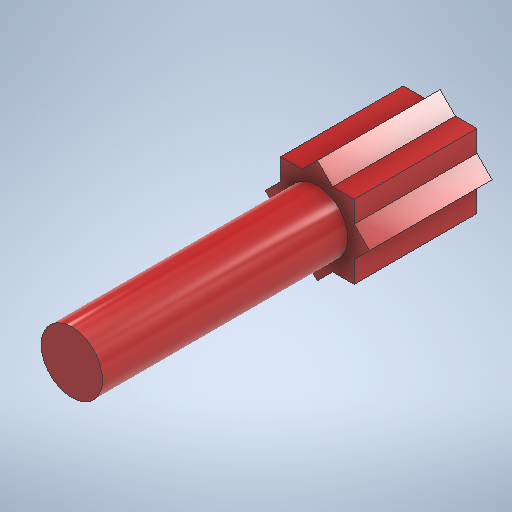
# Autodesk Inventor part: screwhead
Saved by Autodesk Inventor 2025 (Build 290162000, 162)
## iProperties
Created: 2025-05-09
Part Number: screwhead
Material: Generic
Document SubType Name: Modeling
Designer: thesn
Density: 1 g/cm^3
Appearance: Default
Author: thesn
Autodesk Inventor part; units mm, degrees
ref_plane "YZ Plane" through (0, 0, 0) normal (1, 0, 0) x (0, 1, 0)
ref_plane "XZ Plane" through (0, 0, 0) normal (0, 1, 0) x (-1, 0, 0)
ref_plane "XY Plane" through (0, 0, 0) normal (0, 0, 1) x (1, 0, 0)
sketch "Sketch1" plane through (0, 0, 0) normal (0, 0, 1) x (1, 0, 0)
  circle A0 centre (0, 0) radius 0.762
  line L0 (-1.0776, 0) -> (0, 1.0776)
  line L1 (0, 1.0776) -> (1.0776, 0)
  line L2 (1.0776, 0) -> (0, -1.0776)
  line L3 (0, -1.0776) -> (-1.0776, 0)
  line L4 (-0.762, 0.762) -> (0.762, 0.762)
  line L5 (0.762, 0.762) -> (0.762, -0.762)
  line L6 (0.762, -0.762) -> (-0.762, -0.762)
  line L7 (-0.762, -0.762) -> (-0.762, 0.762)
  point P0 (0, 3.175)
  point P1 (-3.175, 0)
  point P2 (-0.898, 0.898)
  point P3 (-0.6286, -0.0898)
  point P4 (-0.5388, -0.5388)
  point P5 (0.5388, -0.5388)
  point P6 (0.3287, 1.2267)
  point P7 (3.7343, 0.7559)
  point P8 (0.5388, 0.5388)
  point P9 (-0.5388, 0.5388)
  point P10 (0, 0.762)
  point P11 (-0.762, 0)
  point P12 (0.3156, 0.762)
  point P13 (-0.3156, 0.762)
  point P14 (-0.762, 0.3156)
  point P15 (-0.762, -0.3156)
  point P16 (-0.3156, -0.762)
  point P17 (0.3156, -0.762)
  point P18 (0.762, -0.3156)
  point P19 (0.762, 0.3156)
  dimension "d0" = 1.524
  dimension "d1" = 1.524
  dimension "d2" = 1.524
  dimension "d3" = 0
  dimension "d12" = 0
  dimension "d13" = 0
  dimension "d16" = 1.524
  dimension "d17" = 1.524
  dimension "d18" = 0
  dimension "d19" = 0
  constraints: 16 end point, 4 parallel, 2 midpoint, 2 perpendicular, 1 centre point, 1 coincident, 1 horizontal
  measures "d0" diameter of A0
  measures "d1" distance of L1.end L2.end
  measures "d2" distance between parallel lines of L2 L0
  measures "d3" horizontal distance of point (0, 0) point (0, 3.175)
  measures "d12" horizontal distance of point (0, 0) L0.end
  measures "d13" vertical distance of point (0, 0) L1.end
  measures "d16" distance of L5.end L6.end
  measures "d17" distance of L4.end L5.end
  measures "d18" horizontal distance of point (0, 0) point (0, 0.762)
  measures "d19" vertical distance of point (0, 0) point (-0.762, 0)
extrude "Extrusion3" add sketch "Sketch1" against normal blind 7.62
sketch "Sketch6" plane through (0, 0, 0) normal (0, 0, 1) x (1, 0, 0)
  line L0 (-0.762, 0.3156) -> (-0.762, 0.762) projected
  circle A0 centre (0, 0) radius 1.0776
  line L1 (-0.762, 0.762) -> (-0.3156, 0.762) projected
  circle A1 centre (0, 0) radius 0.635
  dimension "d33" = 1.27
  constraints: 2 coincident, 1 centre point, 3 other
  measures "d33" diameter of A1
extrude "Extrusion6" cut sketch "Sketch6" against normal blind 5.08
sketch "Sketch7" plane through (0, 0, -7.62) normal (0, 0, -1) x (-1, 0, 0)
  line L0 (-1.6188, 0.635) -> (1.6188, 0.635) construction
  line L1 (1.6188, 0.635) -> (1.6188, -0.635) construction
  line L2 (1.6188, -0.635) -> (-1.6188, -0.635) construction
  line L3 (-1.6188, -0.635) -> (-1.6188, 0.635) construction
  line L4 (-0.1528, -0.1398) -> (-0.1528, -0.2286)
  line L5 (-0.1528, -0.2286) -> (0.0123, -0.2286)
  line L6 (0.0123, -0.2286) -> (0.0123, 0.2282)
  line L7 (0.0123, 0.2282) -> (-0.1657, 0.2282)
  spline S0 degree 2 poles (-0.1657, 0.2282) (-0.2188, 0.2282) (-0.291, 0.1916) (-0.3147, 0.1563) knots 0 0 0 1 2 2 2
  line L8 (-0.3147, 0.1563) -> (-0.5796, -0.2286)
  line L9 (-0.5796, -0.2286) -> (-0.3825, -0.2286)
  line L10 (-0.3825, -0.2286) -> (-0.3258, -0.1398)
  line L11 (-0.3258, -0.1398) -> (-0.1528, -0.1398)
  line L12 (-0.25, -0.0203) -> (-0.1769, 0.0943)
  spline S1 degree 2 poles (-0.1769, 0.0943) (-0.1715, 0.1028) (-0.1608, 0.1091) (-0.1541, 0.1086) knots 0 0 0 1 2 2 2
  line L13 (-0.1541, 0.1086) -> (-0.1528, 0.1086)
  line L14 (-0.1528, 0.1086) -> (-0.1528, -0.0203)
  line L15 (-0.1528, -0.0203) -> (-0.25, -0.0203)
  line L16 (0.0783, 0.1086) -> (0.238, 0.1086)
  line L17 (0.238, 0.1086) -> (0.238, -0.2286)
  line L18 (0.238, -0.2286) -> (0.403, -0.2286)
  line L19 (0.403, -0.2286) -> (0.403, 0.1086)
  line L20 (0.403, 0.1086) -> (0.5627, 0.1086)
  line L21 (0.5627, 0.1086) -> (0.5627, 0.2282)
  line L22 (0.5627, 0.2282) -> (0.0801, 0.2282)
  line L23 (0.0801, 0.2282) -> (0.0783, 0.1086)
  point P0 (0, 0)
  point P1 (0, 0.635)
  point P2 (-1.6188, 0)
  dimension "d34" = 0
  dimension "d35" = 0
  constraints: 2 midpoint, 2 other
  measures "d34" horizontal distance of point (0, 0) point (0, 0.635)
  measures "d35" vertical distance of point (0, 0) point (-1.619, 0)
extrude "Extrusion7" cut sketch "Sketch7" against normal blind 0.508
body "Solid2"
